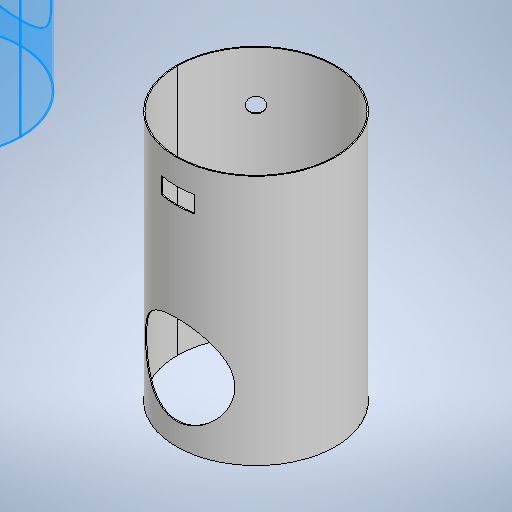
# Autodesk Inventor part: PNS 9110 main Shell D 940
Saved by Autodesk Inventor 2025.3 (Build 293356030, 356C)
## iProperties
Created: 2025-02-11
Part Number: PNS 9110 main Shell D 940
Material: Steel
Document SubType Name: Sheet Metal
Designer: pokla
Mass: 197479 g
Surface Area: 84554.1 cm^2
Volume: 25156.5 cm^3
Density: 7.85 g/cm^3
Flat Pattern Width: 150 cm
Flat Pattern Length: 296.886 cm
Flat Pattern Area: 44532.9 cm^2
Sheet Metal Rule: Default_mm
Sheet Metal Width: 1500,000 mm
Sheet Metal Length: 2968,860 mm
Sheet Metal Area: 4453289,687 mm^2
Appearance: Default
Author: pokla
Autodesk Inventor part; units mm, degrees
ref_plane "YZ Plane" through (0, 0, 0) normal (1, 0, 0) x (0, 1, 0)
ref_plane "XZ Plane" through (0, 0, 0) normal (0, 1, 0) x (-1, 0, 0)
ref_plane "XY Plane" through (0, 0, 0) normal (0, 0, 1) x (1, 0, 0)
sketch "Sketch1" plane through (0, 0, 0) normal (0, 1, 0) x (-1, 0, 0)
  line L0 (476, 1500) -> (470, 1500)
  line L1 (470, 1500) -> (470, 0)
  line L2 (470, 0) -> (476, 0)
  line L3 (476, 0) -> (476, 1500)
  line L4 (0, 0) -> (0, 1673.0415)
  point P0 (473, 0)
  dimension "d0" = 6
  dimension "d1" = 1500
  dimension "d2" = 940
  constraints: 10 end point, 2 parallel, 1 coincident, 1 horizontal, 1 horizontal alignment, 1 midpoint, 1 perpendicular, 1 vertical
  measures "d0" distance between parallel lines of L1 L3
  measures "d1" distance of L2.end L0.start
  measures "d2" diameter of L1 L4
revolve "Revolution1" add sketch "Sketch1" angle 359.9 about axis through (0, 0, 0) along (0, 0, 1)
sketch "Sketch2" plane through (0, 0, 0) normal (0, 1, 0) x (-1, 0, 0)
  circle A0 centre (0, 400) radius 267.5
  line L0 (470, 1500) -> (-470, 1500) projected
  line L1 (110, 1300) -> (-110, 1300) construction
  line L2 (110, 1390) -> (-110, 1390)
  line L3 (-110, 1210) -> (110, 1210)
  arc A1 (110, 1210) -> (110, 1390) centre (110, 1300) ccw
  arc A2 (-110, 1390) -> (-110, 1210) centre (-110, 1300) ccw
  line L4 (200, 1300) -> (-200, 1300) construction
  point P0 (0, 0)
  point P1 (469.9993, 1500)
  point P2 (0, 1300)
  dimension "d4" = 535
  dimension "d12" = 400
  dimension "d15" = 200
  dimension "d16" = 400
  dimension "d17" = 180
  constraints: 10 end point, 6 point on circle, 4 tangent, 3 centre point, 2 vertical alignment, 1 horizontal, 1 midpoint, 1 parallel
  measures "d4" diameter of A0
  measures "d12" distance of A0.centre point (0, 0)
  measures "d15" distance between parallel lines of L1 L0
  measures "d16" distance of L4.start L4.end
  measures "d17" distance between parallel lines of L3 L2
extrude "Extrusion1" cut sketch "Sketch2" against normal through all contours A0
sketch "floor angle sketch" plane through (0, 0, 0) normal (0, 0, 1) x (1, 0, 0)
  line L0 (0, 0) -> (0, -267.717)
  line L1 (0, -267.717) -> (0, 0)
  line L2 (0, 0) -> (0, -172)
  line L3 (0, 0) -> (-63.6396, 63.6396)
  line L4 (0, 0) -> (23.2937, -86.9333)
  dimension "Feeder_way_angle" = 0
  dimension "Feeder_way_line" = 172
  dimension "Outer_way_line" = 90
  dimension "Inner_way_line" = 90
  dimension "Outer_way_angle" = 345
  dimension "Inner_way_angle" = 135
  constraints: 10 end point, 1 collinear, 1 vertical
  measures "Feeder_way_angle" distance between parallel lines of L0 L2
  measures "Feeder_way_line" distance of L0.start L2.end
  measures "Outer_way_line" distance of L0.start L4.end
  measures "Inner_way_line" distance of L0.start L3.end
  measures "Inner_way_angle" angle of L0 L3
ref_plane "Feeder Plane" through (0, 0, -10) normal (1, 0, 0) x (0, 0, 1)
sketch "Feeder horisont hight angle" plane through (0, 0, -10) normal (1, 0, 0) x (0, 0, 1)
  line L0 (1510, -470) -> (1510, 470) construction
  line L1 (10, 0) -> (1510, 0) construction
  line L2 (1310, 0) -> (1310, 476)
  line L3 (10, 476) -> (1510, 476) construction
  line L4 (1310, 476) -> (1310, 0) construction
  point P0 (1510, 0)
  point P1 (1510, -0.8203)
  dimension "d34" = 1300
  dimension "d35" = 0
  constraints: 6 end point, 3 point on line, 1 midpoint, 1 perpendicular
  measures "d34" distance of L3.start L2.end
  measures "d35" distance between parallel lines of L2 L4
ref_plane "Feeder Work Plane" through (0, 0, 1300) normal (0, -1, 0) x (1, 0, 0)
sketch "Sketch8" plane through (0, 0, 1300) normal (0, -1, 0) x (1, 0, 0)
  circle A0 centre (0, 0) radius 86 construction
  line L0 (-100, 50) -> (100, 50)
  line L1 (100, 50) -> (100, -50)
  line L2 (100, -50) -> (-100, -50)
  line L3 (-100, -50) -> (-100, 50)
  line L4 (-100, 50) -> (100, -50) construction
  line L5 (100, 50) -> (-100, -50) construction
  arc A1 (-100, -50) -> (100, -50) centre (0, 409.2385) ccw construction
  arc A2 (-100, 50) -> (100, 50) centre (0, 509.2385) ccw construction
  point P0 (0, -1300)
  point P1 (0, 0)
  dimension "d36" = 172
  dimension "d50" = 200
  dimension "d51" = 100
  dimension "d52" = 470
  constraints: 12 end point, 4 point on circle, 3 centre point, 2 midpoint, 2 parallel, 1 coincident, 1 equal radius, 1 horizontal, 1 perpendicular, 1 vertical alignment
  measures "d36" diameter of A0
  measures "d50" distance of L1.end L2.end
  measures "d51" distance of L0.end L1.end
  measures "d52" radius of A1
extrude "Feeder Extrusion" cut sketch "Sketch8" along normal through all
ref_plane "Inner Plane" through (0, 0, 0) normal (0.7071068, 0.7071068, 0) x (-0.7071068, 0.7071068, 0)
sketch "Inner horisont hight angle" plane through (0, 0, 0) normal (0.7071068, 0.7071068, 0) x (-0.7071068, 0.7071068, 0)
  line L0 (476, 1500) -> (-476, 1500) construction
  line L1 (476, 0) -> (476, 1500) construction
  line L2 (0, 0) -> (0, 1500) construction
  line L3 (0, 1200) -> (476, 1200) construction
  line L4 (476, 1200) -> (0, 1200)
  point P0 (336.5828, 1500)
  point P1 (337.1698, 1500)
  dimension "d40" = 0
  dimension "d41" = 1200
  constraints: 6 end point, 3 point on line, 1 midpoint, 1 perpendicular
  measures "d40" distance between parallel lines of L4 L3
  measures "d41" distance of L1.start L3.end
ref_plane "Inner Work Plane" through (0, 0, 1200) normal (0.7071068, -0.7071068, 0) x (0.7071068, 0.7071068, 0)
sketch "Sketch10" plane through (0, 0, 1200) normal (0.7071068, -0.7071068, 0) x (0.7071068, 0.7071068, 0)
  circle A0 centre (0, 0) radius 45.5
  point P0 (0, -1200)
  point P1 (0, 0)
  point P2 (0, 0)
  point P3 (0, 0)
  dimension "d42" = 91
  constraints: 1 centre point, 1 coincident
  measures "d42" diameter of A0
extrude "Inner Extrusion" cut sketch "Sketch10" against normal through all
ref_plane "Outer Plane" through (0, 0, 0) normal (-0.9659258, -0.258819, 0) x (0.258819, -0.9659258, 0)
sketch "Sketch11" plane through (0, 0, 0) normal (-0.9659258, -0.258819, 0) x (0.258819, -0.9659258, 0)
  line L0 (0, 0) -> (0, 1500)
  line L1 (476, 1500) -> (-476, 1500) projected
  line L2 (0, 700) -> (476, 700)
  line L3 (476, 0) -> (476, 1500) projected
  line L4 (476, 700) -> (0, 700)
  point P0 (-123.1979, 1500)
  point P1 (-124.0001, 1500)
  dimension "d45" = 0
  dimension "d46" = 700
  constraints: 6 end point, 3 point on line, 1 midpoint, 1 perpendicular
  measures "d45" distance between parallel lines of L4 L2
  measures "d46" distance of L3.start L2.end
ref_plane "Work Plane9" through (0, 0, 700) normal (-0.258819, 0.9659258, 0) x (-0.9659258, -0.258819, 0)
sketch "Sketch12" plane through (0, 0, 700) normal (-0.258819, 0.9659258, 0) x (-0.9659258, -0.258819, 0)
  circle A0 centre (0, 0) radius 46
  point P0 (0, -700)
  point P1 (0, 0)
  point P2 (0, 0)
  point P3 (0, 0)
  dimension "d47" = 92
  constraints: 1 centre point, 1 coincident
  measures "d47" diameter of A0
extrude "Extrusion6" [suppressed]
equation "\"d2\" = MAIN_filter_diam"
equation "\"d4\" = Accsess_hatch_diameter"
equation "\"d16\" = Charging_hatch_width"
equation "\"d17\" = Charging_hatch_hight"
equation "\"d34\" = Feedr_hight"
equation "\"BendRadius\" = Thickness"
equation "\"BendReliefWidth\" = Thickness"
equation "\"BendReliefDepth\" = 0.5 * Thickness"
equation "\"CornerReliefSize\" = 4 * Thickness"
equation "\"MinimumRemnant\" = 2 * Thickness"
equation "\"TransitionRadius\" = BendRadius"
equation "\"JacobiRadiusSize\" = BendRadius"
equation "\"GapSize\" = Thickness"
equation "\"Feedr_hight\" = 1300"
equation "\"Feeder_horisont_hight_angle\" = 0"
equation "\"MAIN_filter_diam\" = 940"
equation "\"Accsess_hatch_diameter\" = 535"
equation "\"Charging_hatch_width\" = 400"
equation "\"Charging_hatch_hight\" = 180"
equation "\"Thickness\" = 6"
body "Solid1"
